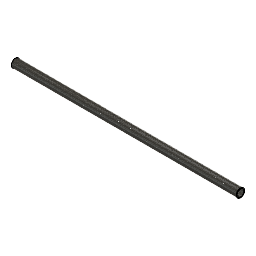
cad_native (Autodesk Fusion 360 archive; units mm, degrees)
design "Carbon fibre pipe"
Autodesk Fusion 360 part; units mm, degrees
note: some values were not read from the file. Chosen so that the rebuilt part matches the saved one: which face or edge a step refers to; how an offset face is resized.
sketch "Sketch1" plane through (0, 0, 0) normal (1, 0, 0) x (0, 0, -1)
  circle A0 centre (0, 0) radius 5
  circle A1 centre (0, 0) radius 6
  dimension "d1" = 10
  dimension "d2" = 12
  constraint coincident A0.centre A1.centre
  measures "d1" diameter of A0
  measures "d2" diameter of A1
extrude "Extrude1" add sketch "Sketch1" along normal blind 320

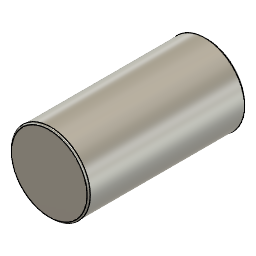
design "15mm by 20mm axial magnet"
Autodesk Fusion 360 part; units mm, degrees
sketch "Sketch1" plane through (0, 0, 0) normal (0, 0, 1) x (1, 0, 0)
  circle A0 centre (0, 0) radius 5
  dimension "d1" = 10
  constraint coincident A0.centre origin
  measures "d1" diameter of A0
extrude "Extrude1" add sketch "Sketch1" along normal blind 20
fillet "Fillet1" radius 0.2 2 edges at (-4.6616, -1.8081, 20) (-4.6616, -1.8081, 0)

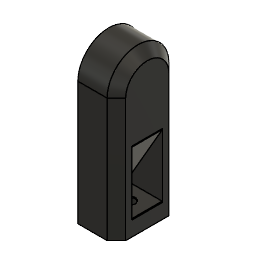
design "stator_holders"
Autodesk Fusion 360 part; units mm, degrees
sketch "Base" plane through (0, 0, 0) normal (1, 0, 0) x (0, 0, -1)
  circle A0 centre (0, 0) radius 6.1
  circle A1 centre (0, 0) radius 10 construction
  line L0 (0, 0) -> (-10, 0) construction
  line L1 (0, 0) -> (0, -40) construction
  line L2 (0, -40) -> (-10, -40)
  line L3 (-10, -40) -> (-10, 0)
  line L4 (10, -40) -> (10, 0)
  line L5 (0, -40) -> (10, -40)
  line L6 (0, 0) -> (0, 10) construction
  arc A2 (10, 0) -> (-10, 0) centre (0, 0) ccw
  dimension "d1" = 12.2
  dimension "d2" = 20
  dimension "d3" = 40
  dimension "d4" = 10
  constraint coincident A0.centre A1.centre
  constraint concentric A0 A1
  constraint coincident A1 L0.end
  constraint horizontal L0
  constraint perpendicular L0 L1
  constraint perpendicular L1 L2
  constraint symmetric L0.end L1 L4.end
  constraint symmetric L2.start L1 L5.start
  constraint symmetric L1 L2.end L4.start
  constraint coincident A1 L6.end
  constraint perpendicular L0 L6
  constraint coincident L6.end A2
  measures "d1" diameter of A0
  measures "d2" diameter of A1
  measures "d3" distance of A0.centre L1.end
  measures "d4" distance of L1.end L2.end
extrude "Extrude1" add sketch "Base" along normal blind 12.5 contours A0 | L2 L3 L4 L5 A2
extrude "Extrude2" cut sketch "Base" along normal blind 10 contours A0
chamfer "Chamfer1" distance 3 angle 45 3 edges at (12.5, 10, 0) (12.5, -20, 10) (12.5, -20, -10)
ref_plane "WorkPlane1" through (6.25, -20, 0) normal (0, 0, -1) x (0, 1, 0)
sketch "Bolt" plane through (0, 0, 0) normal (0, 0, -1) x (0, 1, 0)
  line L0 (0, 0) -> (-30, 0) construction
  line L1 (-30, 0) -> (-30, 12.5) construction
  line L2 (-30, 12.5) -> (0, 12.5) construction
  line L3 (0, 12.5) -> (0, 0) construction
  line L4 (-30, 12.5) -> (-35, 12.5) construction
  line L5 (-35, 12.5) -> (-35, 0) construction
  line L6 (-35, 12.5) -> (-35, 2.5)
  line L7 (-35, 2.5) -> (-32, 2.5)
  line L8 (-32, 2.5) -> (-14.6795, 12.5)
  line L9 (-35, 12.5) -> (-14.6795, 12.5)
  dimension "d11" = 12.5
  dimension "d12" = 10
  dimension "d13" = 20
  constraint horizontal L0
  constraint vertical L1
  constraint horizontal L2
  constraint vertical L3
  constraint coincident L0.start L3.end
  constraint coincident L2 L4.end
  constraint coincident L0 L5.end
  constraint perpendicular L0 L5
  constraint perpendicular L2 L6
  constraint perpendicular L6 L7
  constraint coincident L2 L8.end
  measures "d11" distance of L0.start L2.end
  measures "d12" distance of L4.end L6.end
  measures "d13" distance of L7.end L8.end
extrude "Extrude3" cut sketch "Bolt" along normal blind 5
extrude "Extrude4" cut 1 faces at (9.1667, -27.2265, 0) along direction (0, 0, 1) blind 5
sketch "Sketch3" plane through (0, -35, 0) normal (0, 1, 0) x (-1, 0, 0)
  line L0 (-12.5, 5) -> (-12.5, -5)
  line L1 (-12.5, -5) -> (-2.5, -5)
  line L2 (-2.5, -5) -> (-2.5, 5)
  line L3 (-2.5, 5) -> (-12.5, 5)
  line L4 (-12.5, 5) -> (-2.5, 5)
  line L5 (-2.5, 5) -> (-2.5, -5)
  line L6 (-2.5, -5) -> (-12.5, -5)
  line L7 (-12.5, -5) -> (-12.5, 5)
  circle A0 centre (-7, 0) radius 1.5
  dimension "d18" = 3
  constraint horizontal L4
  constraint vertical L5
  constraint horizontal L6
  constraint vertical L7
  constraint coincident L1.end L2.start
  constraint coincident L0.start L3.end
  measures "d18" diameter of A0
extrude "Extrude5" cut sketch "Sketch3" against normal blind 6 contours A0
chamfer "Chamfer2" distance 0.2 angle 45 1 edges at (8.3985, -35, 0.5424)
chamfer "Chamfer3" distance 0.2 angle 45 4 edges at (2.5, -35, 0) (2.5, -32, 0) (12.5, -14.6795, 0) (12.5, -35, 0)
chamfer "Chamfer4" distance 0.3 angle 45 1 edges at (0, -2.2059, 5.6872)

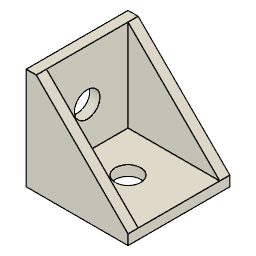
design "Aluminium connections"
Autodesk Fusion 360 part; units mm, degrees
sketch "Base & hole" plane through (0, 0, 0) normal (0, 1, 0) x (1, 0, 0)
  line L0 (0, 0) -> (20, 0)
  line L1 (20, 0) -> (20, 20)
  line L2 (20, 20) -> (0, 20)
  line L3 (0, 20) -> (0, 0)
  circle A0 centre (10, 10) radius 2.5
  dimension "d1" = 20
  dimension "d2" = 20
  dimension "d3" = 5
  constraint horizontal L0
  constraint vertical L1
  constraint horizontal L2
  constraint vertical L3
  constraint coincident L0.start L3.end
  measures "d1" distance of L0.start L0.end
  measures "d2" distance of L0.start L2.end
  measures "d3" diameter of A0
extrude "Extrude1" add sketch "Base & hole" along normal blind 20
sketch "Top" plane through (0, 20, 0) normal (0, 1, 0) x (-1, 0, 0)
  circle A0 centre (-10, -10) radius 2.5
  line L0 (0, -20) -> (0, 0)
  line L1 (0, 0) -> (-20, 0)
  line L2 (-20, 0) -> (-20, -20)
  line L3 (-20, -20) -> (0, -20)
  line L4 (-20, -20) -> (-20, -18) construction
  line L5 (-20, -18) -> (-2, -18)
  line L6 (-2, -18) -> (-2, -2)
  line L7 (-2, -2) -> (-20, -2)
  dimension "d6" = 2
  dimension "d7" = 18
  dimension "d8" = 16
  constraint coincident L2.end L3.start
  constraint perpendicular L3 L4
  constraint perpendicular L0 L5
  constraint perpendicular L3 L6
  constraint coincident L2 L7.end
  constraint perpendicular L2 L7
  measures "d6" distance of L2.end L4.end
  measures "d7" distance of L4.end L5.end
  measures "d8" distance of L5.end L6.end
extrude "Extrude2" cut sketch "Top" against normal blind 18 contours L2 L5 L6 L7
sketch "Side removal" plane through (0, 0, 0) normal (0, 0, 1) x (1, 0, 0)
  line L0 (0, 0) -> (20, 0)
  line L1 (20, 0) -> (20, 20)
  line L2 (20, 20) -> (0, 20)
  line L3 (0, 20) -> (0, 0)
  line L4 (0, 20) -> (2, 20)
  line L5 (20, 0) -> (20, 2)
  line L6 (20, 2) -> (2, 20)
  dimension "d11" = 2
  dimension "d12" = 2
  constraint coincident L2.end L3.start
  constraint perpendicular L3 L4
  constraint coincident L0.end L1.start
  constraint perpendicular L0 L5
  measures "d11" distance of L2.end L4.end
  measures "d12" distance of L0.end L5.end
extrude "Extrude3" cut sketch "Side removal" against normal blind 30 contours L1 L2 L6
sketch "side hole" plane through (0, 0, 0) normal (-1, 0, 0) x (0, 0, 1)
  line L0 (-20, 0) -> (0, 0)
  line L1 (0, 0) -> (0, 20)
  line L2 (0, 20) -> (-20, 20)
  line L3 (-20, 20) -> (-20, 0)
  circle A0 centre (-10, 10) radius 2.5
  dimension "d15" = 5
  measures "d15" diameter of A0
extrude "Extrude4" cut sketch "side hole" against normal blind 5 contours A0

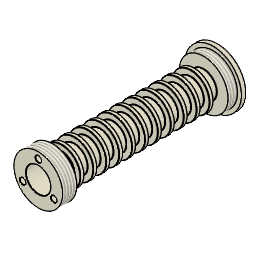
design "Armature core"
Autodesk Fusion 360 part; units mm, degrees
sketch "Armature Base" plane through (0, 0, 0) normal (0, 0, 1) x (1, 0, 0)
  circle A0 centre (0, 0) radius 10
  circle A1 centre (0, 0) radius 6.5
  dimension "d1" = 20
  dimension "d2" = 13
  constraint coincident A0.centre A1.centre
  measures "d1" diameter of A0
  measures "d2" diameter of A1
extrude "Extrude1" add sketch "Armature Base" along normal blind 95
ref_plane "WorkPlane2" through (0, 0, 7.5) normal (0, 0, -1) x (-1, 0, 0)
sketch "Slot Base" plane through (0, 0, 7.5) normal (0, 0, -1) x (-1, 0, 0)
  circle A0 centre (0, 0) radius 7
  circle A1 centre (0, 0) radius 10
  dimension "d33" = 14
  dimension "d34" = 20
  constraint coincident A0.centre A1.centre
  constraint concentric A0 A1
  measures "d33" diameter of A0
  measures "d34" diameter of A1
extrude "Extrude6" cut sketch "Slot Base" against normal blind 4.8333
fillet "Fillet2" radius 0.2 2 edges at (6.5263, 2.5313, 7.5) (6.5263, -2.5313, 12.3333)
pattern_linear "R-Pattern3" count 12 spacing 6.8333 along (0, 0, 1) of 5 faces at (-6.9913, -0.3489, 10.6556) (4.0943, -5.6948, 12.2064) (9.0026, 0.8545, 12.3333) (-6.1569, -3.3529, 7.6357) (9.0026, 0.8545, 7.5)
sketch "Extend Base" plane through (0, 0, 0) normal (0, 0, -1) x (-1, 0, 0)
  circle A0 centre (0, 0) radius 6.5
  circle A1 centre (0, 0) radius 10
  circle A2 centre (0, 0) radius 15
  dimension "d47" = 30
  constraint coincident A0.centre A1.centre
  measures "d47" diameter of A2
extrude "Extrude7" add sketch "Extend Base" against normal blind 7.5 contours A2
sketch "Extend Base 2" plane through (0, 0, 95) normal (0, 0, 1) x (1, 0, 0)
  circle A0 centre (0, 0) radius 6.5
  circle A1 centre (0, 0) radius 10
  circle A2 centre (0, 0) radius 13
  circle A3 centre (0, 0) radius 6.5
  constraint concentric A0 A2
  constraint concentric A0 A3
sketch "Screw threads" plane through (0, 0, 7.5) normal (0, 0, 1) x (1, 0, 0)
  circle A0 centre (0, 0) radius 15
  circle A1 centre (0, 0) radius 7.2
  circle A2 centre (0, 0) radius 13
  circle A3 centre (0, 0) radius 15
  constraint concentric A0 A2
  constraint concentric A2 A3
extrude "Extrude8" cut sketch "Screw threads" against normal blind 5 contours A0 A3
extrude "Extrude9" add sketch "Extend Base 2" against normal blind 7.5 contours A2
fillet "Fillet3" radius 0.2 22 edges at (-9.3233, -3.6162, 12.3333) (-9.3233, -3.6162, 14.3333) (-9.3233, 3.6162, 19.1667) (-9.3233, -3.6162, 21.1667) (-9.3233, 3.6162, 26) (-9.3233, -3.6162, 28) (-9.3233, 3.6162, 32.8333) (-9.3233, -3.6162, 34.8333) (-9.3233, 3.6162, 39.6667) (-9.3233, -3.6162, 41.6667) (-9.3233, 3.6162, 46.5) (-9.3233, -3.6162, 48.5) (-9.3233, 3.6162, 53.3333) (-9.3233, -3.6162, 55.3333) (-9.3233, 3.6162, 60.1667) (-9.3233, -3.6162, 62.1667) (-9.3233, 3.6162, 67) (-9.3233, -3.6162, 69) (-9.3233, 3.6162, 73.8333) (-9.3233, -3.6162, 75.8333) (-9.3233, 3.6162, 80.6667) (-9.3233, -3.6162, 82.6667)
thread "Thread1" "ISO Metric profile 26.0 M26x1.5 M26x1.5 6g" major diameter 25.85 minor diameter 24.1319 pitch 1.5 angle 60 resizes the face on face at (12.9838, -0.648, 4.1667)
sketch "120 deg screw holes" plane through (0, 0, 0) normal (0, 0, -1) x (-1, 0, 0)
  circle A0 centre (0, 0) radius 15
  circle A1 centre (0, 0) radius 6.5
  line L0 (0, 0) -> (0, 9.5) construction
  circle A2 centre (0, 9.5) radius 1.5
  line L1 (0, 0) -> (-8.2272, -4.75) construction
  line L2 (0, 0) -> (-9.5, 0) construction
  circle A3 centre (-8.2272, -4.75) radius 1.5
  line L3 (0, 0) -> (8.2272, -4.75) construction
  line L4 (0, 0) -> (9.5, 0) construction
  circle A4 centre (8.2272, -4.75) radius 1.5
  dimension "d58" = 9.5
  dimension "d59" = 3
  dimension "d60" = 30
  dimension "d61" = 9.5
  dimension "d62" = 3
  dimension "d63" = 30
  dimension "d64" = 9.5
  dimension "d65" = 3
  constraint coincident A0.centre A1.centre
  constraint vertical L0
  constraint coincident L0.end A2.centre
  constraint horizontal L2
  constraint coincident L1.end A3.centre
  constraint horizontal L4
  constraint coincident L3.end A4.centre
  measures "d58" distance of A0.centre L0.end
  measures "d59" diameter of A2
  measures "d60" angle of L1 L2
  measures "d61" distance of A0.centre L1.end
  measures "d62" diameter of A3
  measures "d63" angle of L3 L4
  measures "d64" distance of A0.centre L3.end
  measures "d65" diameter of A4
extrude "Extrude10" cut sketch "120 deg screw holes" against normal blind 5 contours A2 | A3 | A4
ref_plane "WorkPlane3" through (0, 0, 47.5) normal (0, 0, -1) x (-1, 0, 0)
fillet "Fillet4" radius 0.2 4 edges at (1.3985, 10.0424, 0) (9.6257, -4.2076, 0) (-6.8288, -4.2076, 0) (13.9849, -5.4242, 0)
fillet "Fillet4" radius 0.2 1 edges at (-6.0601, 2.3505, 0)
fillet "Fillet4" radius 0.2 1 edges at (-6.0601, 2.3505, 95)
mirror "Mirror1" about plane through (0, 0, 47.5) normal (0, 0, -1) of 9 faces at (0.7712, 7.9957, 0.0002) (-1.4981, 9.4252, 3.4) (9.785, -5.4066, 0.0002) (6.7291, -4.8248, 3.4) (-9.785, -5.4066, 0.0002) (-9.7254, -4.8248, 3.4) (0.1827, 9.9654, 5) (8.9417, -4.6423, 5) (-7.6015, -4.9661, 5)
thread "Thread2" "ISO Metric profile 26.0 M26x1.5 M26x1.5 6g" major diameter 25.85 minor diameter 24.1319 pitch 1.5 angle 60 resizes the face on face at (12.9838, -0.648, 92.5)
equation "d32 = -6 mm - 1.5 mm"
equation "d45 = 4.833333333 mm + 2 mm"

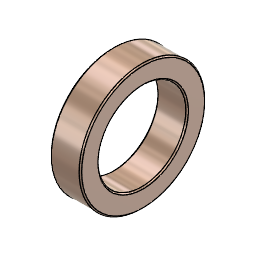
design "coil"
Autodesk Fusion 360 part; units mm, degrees
sketch "Sketch10" plane through (0, 0, 0) normal (1, 0, 0) x (0, 0, -1)
  circle A0 centre (0, 0) radius 7
  circle A1 centre (0, 0) radius 10
  dimension "d34" = 14
  dimension "d35" = 20
  constraint coincident A0.centre A1.centre
  constraint concentric A0 A1
  measures "d34" diameter of A0
  measures "d35" diameter of A1
extrude "Extrude3" add sketch "Sketch10" along normal blind 4.8333
fillet "Fillet2" radius 0.2 4 edges at (4.8333, 2.5313, 6.5263) (4.8333, -3.6162, 9.3233) (0, 2.5313, 6.5263) (0, -3.6162, 9.3233)

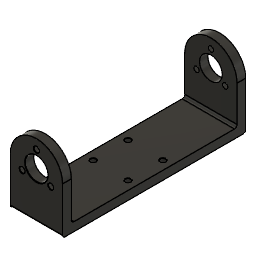
design "armature holder"
Autodesk Fusion 360 part; units mm, degrees
sketch "Base" plane through (0, 0, 0) normal (0, 0, 1) x (1, 0, 0)
  line L0 (0, 0) -> (15, 0) construction
  line L1 (0, 0) -> (8.2272, -4.75) construction
  line L2 (0, 0) -> (-9.5, 0) construction
  circle A0 centre (8.2272, -4.75) radius 1.5
  circle A1 centre (0, 9.5) radius 1.5
  circle A2 centre (-8.2272, -4.75) radius 1.5
  circle A3 centre (0, 0) radius 15 construction
  line L3 (0, 0) -> (0, -27) construction
  line L4 (0, -27) -> (15, -27)
  line L5 (15, -27) -> (15, 0)
  line L6 (-15, -27) -> (-15, 0)
  line L7 (0, -27) -> (-15, -27)
  line L8 (0, 0) -> (0, 15) construction
  arc A4 (15, 0) -> (-15, 0) centre (0, 0) ccw
  circle A5 centre (0, 0) radius 6.5
  dimension "d1" = 15
  dimension "d2" = 150
  dimension "d3" = 9.5
  dimension "d4" = 3
  dimension "d6" = 360
  dimension "d7" = 27
  dimension "d25" = 13
  constraint coincident L0.start L1.start
  constraint horizontal L0
  constraint horizontal L2
  constraint coincident L1.end A0.centre
  constraint coincident L0.end A3
  constraint perpendicular L0 L3
  constraint perpendicular L3 L4
  constraint tangent A3 L5
  constraint symmetric L0.end L3 L6.end
  constraint symmetric L4.start L3 L7.start
  constraint symmetric L3 L4.end L6.start
  constraint coincident A3 L8.end
  constraint parallel L3 L8
  constraint coincident L8.end A4
  constraint concentric A4 A5
  measures "d1" distance of L0.start L0.end
  measures "d2" angle of L1 L2
  measures "d3" distance of L0.start L1.end
  measures "d4" diameter of A0
  measures "d7" distance of L0.start L3.end
  measures "d25" diameter of A5
extrude "Extrude1" add sketch "Base" along normal blind 105
ref_plane "WorkPlane1" through (0, 15, 0) normal (0, 1, 0) x (0, 0, 1)
sketch "cutout" plane through (0, 15, 0) normal (0, 1, 0) x (1, 0, 0)
  line L0 (0, 0) -> (15, 0)
  line L1 (15, 0) -> (15, -105)
  line L2 (15, -105) -> (-15, -105)
  line L3 (-15, -105) -> (-15, 0)
  line L4 (-15, 0) -> (-15, -5)
  line L5 (-15, -5) -> (15, -5)
  line L6 (15, -105) -> (15, -100)
  line L7 (15, -100) -> (-15, -100)
  dimension "d11" = 15
  dimension "d12" = 5
  dimension "d13" = 5
  constraint coincident L0.start origin
  constraint horizontal L0
  constraint perpendicular L0 L1
  constraint perpendicular L1 L2
  constraint perpendicular L2 L3
  constraint perpendicular L2 L4
  constraint perpendicular L4 L5
  constraint perpendicular L5 L6
  constraint coincident L3 L7.end
  constraint perpendicular L3 L7
  measures "d11" distance of L0.start L0.end
  measures "d12" distance of L3.end L4.end
  measures "d13" distance of L1.end L6.end
extrude "Extrude2" cut sketch "cutout" against normal blind 37 contours L1 L3 L5 L7
fillet "Fillet1" radius 1.5 4 edges at (0, -22, 100) (0, -22, 5) (0, -27, 105) (0, -27, 0)
sketch "Sketch3" plane through (0, -22, 0) normal (0, 1, 0) x (-1, 0, 0)
  line L0 (-15, 6.5) -> (15, 6.5)
  line L1 (15, 6.5) -> (15, 98.5)
  line L2 (15, 98.5) -> (-15, 98.5)
  line L3 (-15, 98.5) -> (-15, 6.5)
  line L4 (-15, 98.5) -> (-15, 6.5) construction
  line L5 (-15, 52.5) -> (15, 52.5) construction
  line L6 (0, 52.5) -> (0, 62.5) construction
  line L7 (0, 62.5) -> (-10, 62.5) construction
  circle A0 centre (-10, 62.5) radius 1.5
  circle A1 centre (10, 62.5) radius 1.5
  circle A2 centre (-10, 42.5) radius 1.5
  circle A3 centre (10, 42.5) radius 1.5
  dimension "d18" = 10
  dimension "d19" = 10
  dimension "d20" = 3
  constraint coincident L2.end L3.start
  constraint coincident L0.start L3.end
  constraint midpoint L3 L5.start
  constraint midpoint L1 L5.end
  constraint midpoint L5 L6.start
  constraint perpendicular L5 L6
  constraint perpendicular L6 L7
  constraint coincident L7.end A0.centre
  constraint symmetric L6 A0 A1
  constraint symmetric L5 A0 A2
  constraint symmetric L5 A1 A3
  measures "d18" distance of L6.start L6.end
  measures "d19" distance of L6.end L7.end
  measures "d20" diameter of A0
extrude "Extrude3" cut sketch "Sketch3" against normal blind 5 contours A0 | A1 | A2 | A3
chamfer "Chamfer1" distance 0.2 angle 45 4 edges at (11.3985, -22, 63.0424) (11.3985, -22, 43.0424) (-8.6015, -22, 43.0424) (-8.6015, -22, 63.0424)
chamfer "Chamfer2" distance 0.2 angle 45 6 edges at (-1.3985, 10.0424, 0) (6.8288, -4.2076, 0) (-9.6257, -4.2076, 0) (6.8288, -4.2076, 105) (-9.6257, -4.2076, 105) (-1.3985, 10.0424, 105)
chamfer "Chamfer2" distance 0.2 angle 45 2 edges at (-6.0601, 2.3505, 105) (-6.0601, 2.3505, 0)
equation "d7 = 40 mm - 13 mm"
